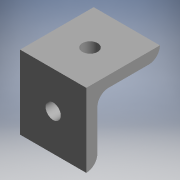
# Autodesk Inventor part: 40-4302 Aluminum
Saved by Autodesk Inventor 2017.3 (Build 213256000, 256)
## iProperties
Part Number: 40-4302 Aluminum
Material: Generic
Catalog Web Link: www.cadenas.de
Description: 25-4119, 40-4302, 20-4119, 30-4302, 45-4302, 30-4302-Black 25-4119-Black, 40-4302-Black, 20-4119-Black, 45-4302-Black-2 Hole Inside Corner Bracket
Vendor: 8020
Document SubType Name: Modeling
Designer: partserver
Manufacturer: 8020
Mass: 15.0566 g
Surface Area: 64.509 cm^2
Volume: 15.0566 cm^3
Density: 1 g/cm^3
Appearance: PSOLRGB-191-191-191
Category: PARTsolutions
Company: 8020
Title: 40-4302
Author: Cadenas PARTsolutions
Comments: 2 Hole Inside Corner Bracket
PSOL_IDENT_0: {$CADENAS_DATA\23d-libs\8020\metric\joining_plates\25_4119.prj},265 {VTYP=3D},{NB=40-4302},{LINA=40-
PSOL_IDENT_1: 4302},{NN=25-4119, 40-4302, 20-4119, 30-4302, 45-4302, 30-4302-Black 25-4119-Black, 40-4302-Black, 2
PSOL_IDENT_2: 0-4119-Black, 45-4302-Black},{DATE=31.07.2020 09:21:28},{GEOMDATE=07.01.2019 15:52:00},{VERSION=},{L
PSOL_IDENT_3: INEID=20},{WBVAR=},{WBNUMERIC=}  {NB=40-4302},{LINA=40-4302},{KT=DUMMY},{PN=40-4302},{SERIES=40},{MA
PSOL_IDENT_4: TERIAL=Aluminum},{GRADE=6105-T5},{FINISH=Clear Anodize},{A=36.00},{B=40.00},{C=40.00},{D=6.00},{E=8.
PSOL_IDENT_5: 30},{W=.039},{D1=6.00000},{R=6.000},{COLOR=.75,.75,.75}
NB: 40-4302
NN: 25-4119, 40-4302, 20-4119, 30-4302, 45-4302, 30-4302-Black 25-4119-Black, 40-4302-Black, 20-4119-Black, 45-4302-Black
NT: 2 Hole Inside Corner Bracket
NBSYN: $PN.
LINA: 40-4302
CATALOG: 80/20
PN: 40-4302
SERIES: 40
MATERIAL: Aluminum
GRADE: 6105-T5
FINISH: Clear Anodize
A: 36
B: 40
C: 40
D: 6
E: 8.3
W: .039
SUPPLIER: 8020
ARTICLENO: 40-4302
BOMINFO: 40-4302
CREATOR: CADENAS GmbH
Autodesk Inventor part; units mm, degrees
ref_plane "YZ Plane" through (0, 0, 0) normal (1, 0, 0) x (0, 1, 0)
ref_plane "XZ Plane" through (0, 0, 0) normal (0, 1, 0) x (-1, 0, 0)
ref_plane "XY Plane" through (0, 0, 0) normal (0, 0, 1) x (1, 0, 0)
sketch "Sketch_1" plane through (0, 0, 0) normal (1, 0, 0) x (0, 1, 0)
  line L0 (0, 40) -> (0, 0)
  line L1 (0, 0) -> (40, 0)
  arc A0 (40, 0) -> (34, 6) centre (34, 0) ccw
  line L2 (34, 6) -> (12, 6)
  arc A1 (6, 12) -> (12, 6) centre (12, 12) ccw
  line L3 (6, 12) -> (6, 34)
  arc A2 (6, 34) -> (0, 40) centre (0, 34) ccw
  constraints: 8 end point, 6 point on circle, 3 centre point
extrude "Extrusion1" add sketch "Sketch_1" along normal mid plane 36
sketch "Sketch2" plane through (18, 40, 0) normal (0, 0, -1) x (-1, 0, 0)
  point P0 (18, -20)
hole "Hole1" at (0, 20, 0) direction (0, 0, 1) diameter 8.3 depth 6
sketch "Sketch3" plane through (-18, 0, 0) normal (0, -1, 0) x (1, 0, 0)
  point P0 (18, 20)
hole "Hole2" at (0, 0, 20) direction (0, 1, 0) diameter 8.3 depth 6
body "Solid1"
